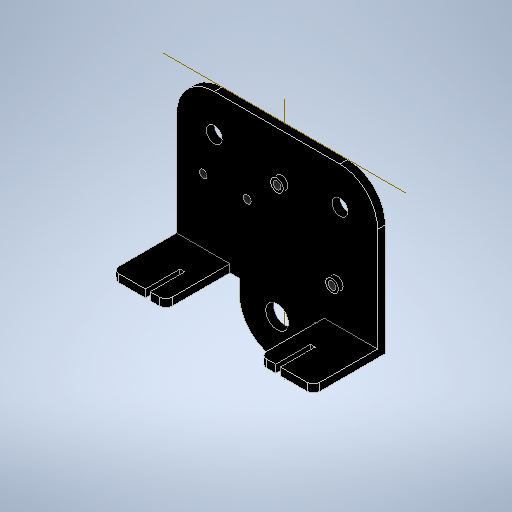
# Autodesk Inventor part: Extruder Plate
Saved by Autodesk Inventor 2025 (Build 290162000, 162)
## iProperties
Manager: J. Wilburn
Created: 2025-03-12
Part Number: Extruder Plate
Material: Aluminum 6061
Document SubType Name: Modeling
Designer: MAL16204
Density: 2.7 g/cm^3
Appearance: Anodized - Black
Mass: 26.6308 g
Surface Area: 91.3048 cm^2
Volume: 9.86327 cm^3
Author: Richard Malstrom
Title: Extruder Plate
Subject: Ender 3 Pro Assembly
Autodesk Inventor part; units mm, degrees
ref_plane "YZ Plane" through (0, 0, 0) normal (1, 0, 0) x (0, 1, 0)
ref_plane "XZ Plane" through (0, 0, 0) normal (0, 1, 0) x (-1, 0, 0)
ref_plane "XY Plane" through (0, 0, 0) normal (0, 0, 1) x (1, 0, 0)
sketch "Sketch1" plane through (0, 0, 0) normal (0, 0, 1) x (1, 0, 0)
  line L0 (-20, 0) -> (20, 0)
  line L1 (32, -12) -> (32, -47.5)
  line L2 (0, -64) -> (0, -64)
  line L3 (-32, -47.5) -> (-32, -12)
  arc A0 (-20, 0) -> (-32, -12) centre (-20, -12) ccw
  arc A1 (32, -12) -> (20, 0) centre (20, -12) ccw
  line L4 (-12, -52) -> (-12, -47.5)
  line L5 (-12, -47.5) -> (-32, -47.5)
  line L6 (12, -52) -> (12, -47.5)
  line L7 (12, -47.5) -> (32, -47.5)
  circle A2 centre (0, -52.1) radius 3.6
  line L8 (0, -80.2794) -> (0, 16.2794) projected
  arc A3 (-12, -52) -> (0, -64) centre (0, -52) ccw
  arc A4 (0, -64) -> (12, -52) centre (0, -52) ccw
  point P0 (0, 0)
  point P1 (0, 0)
  point P2 (0, -64)
  dimension "d0" = 64
  dimension "d1" = 64
  dimension "d2" = 12
  dimension "d3" = 47.5
  dimension "d4" = 47.5
  dimension "d5" = 7.2
  dimension "d6" = 52.1
  dimension "d8" = 12
  dimension "d9" = 12
  dimension "d10" = 12
  constraints: 16 end point, 8 point on circle, 8 tangent, 5 centre point, 2 equal radius, 2 parallel, 1 coincident, 1 horizontal, 1 midpoint, 1 perpendicular, 1 point on line
  measures "d0" distance from line of point (0, 0) L2
  measures "d1" distance between parallel lines of L1 L3
  measures "d2" radius of A0
  measures "d3" distance between parallel lines of L0 L5
  measures "d4" distance between parallel lines of L0 L7
  measures "d5" diameter of A2
  measures "d6" distance of point (0, 0) A2.centre
  measures "d8" distance between parallel lines of L8 L4
  measures "d9" distance between parallel lines of L6 L8
  measures "d10" radius of A3
extrude "Extrusion1" add sketch "Sketch1" along normal blind 2.5 contours L0 L8 A2 A3 L4 L5 L3 A0 | L0 A1 L1 L7 L6 A4 L8 A2
sketch "Sketch2" plane through (0, 0, 2.5) normal (0, 0, 1) x (1, 0, 0)
  line L0 (-32, -47.5) -> (-15, -47.5)
  line L1 (-15, -47.5) -> (-15, -45)
  line L2 (-15, -45) -> (-32, -45)
  line L3 (-32, -45) -> (-32, -47.5)
  line L4 (32, -47.5) -> (32, -12) projected
  line L5 (32, -47.5) -> (15, -47.5)
  line L6 (15, -47.5) -> (15, -45)
  line L7 (15, -45) -> (32, -45)
  line L8 (32, -45) -> (32, -47.5)
  point P0 (0, 0)
  point P1 (-12, -47.5)
  point P2 (12, -47.5)
  point P3 (32, -45)
  point P4 (15, -46.25)
  point P5 (-15, -46.25)
  dimension "d13" = 2.5
  dimension "d17" = 30
  dimension "d18" = 2.5
  constraints: 16 end point, 4 parallel, 2 horizontal, 2 midpoint, 2 perpendicular, 1 collinear, 1 point on line
  measures "d13" distance of L1.end L0.end
  measures "d17" distance of point (15, -46.25) point (-15, -46.25)
  measures "d18" distance between parallel lines of L5 L7
extrude "Extrusion2" add sketch "Sketch2" along normal blind 20.4
sketch "Sketch3" plane through (15, -45, 2.5) normal (0, 1, 0) x (1, 0, 0)
  line L0 (0, -20.4) -> (17, -20.4) projected
  line L1 (6.5, -20.4) -> (5, -20.4)
  line L2 (5, -20.4) -> (5, -9.4)
  line L3 (5, -9.4) -> (6.5, -9.4)
  line L4 (6.5, -9.4) -> (6.5, -20.4)
  line L5 (-3, 2.5) -> (17, 2.5) projected
  line L6 (-30, -20.4) -> (-47, -20.4) projected
  line L7 (-35, -20.4) -> (-36.5, -20.4)
  line L8 (-36.5, -20.4) -> (-36.5, -9.4)
  line L9 (-36.5, -9.4) -> (-35, -9.4)
  line L10 (-35, -9.4) -> (-35, -20.4)
  line L11 (-47, 2.5) -> (-27, 2.5) projected
  line L12 (0, 0) -> (0, -20.4) projected
  point P0 (-15, 2.5)
  point P1 (5, -14.9)
  point P2 (5, -20.4)
  dimension "d19" = 1.5
  dimension "d20" = 11.9
  dimension "d21" = 1.5
  dimension "d22" = 11.9
  dimension "d23" = 40
  dimension "d24" = 5
  constraints: 16 end point, 4 parallel, 2 horizontal, 2 perpendicular, 2 point on line, 1 midpoint
  measures "d19" distance of L2.end L3.end
  measures "d20" distance between parallel lines of L5 L3
  measures "d21" distance of L8.end L9.end
  measures "d22" distance between parallel lines of L11 L9
  measures "d23" distance between parallel lines of L10 L2
  measures "d24" distance from line of L12 point (5, -14.9)
extrude "Extrusion3" cut sketch "Sketch3" against normal through all
fillet "Fillet1" radius 2 4 edges at (32, -46.25, 22.9) (15, -46.25, 22.9) (-15, -46.25, 22.9) (-32, -46.25, 22.9)
sketch "Sketch4" plane through (0, 0, 0) normal (0, 0, -1) x (-1, 0, 0)
  line L0 (-20, 0) -> (20, 0) projected
  line L1 (-32, -47.5) -> (-32, -12) projected
  line L2 (0, -76.8) -> (0, 12.8) projected
  point P0 (0, 0)
  point P1 (-20, -11.9)
  point P2 (20, -11.9)
  dimension "d28" = 11.9
  dimension "d30" = 20
  dimension "d31" = 20
  constraints: 1 horizontal alignment
  measures "d28" distance from line of L0 point (-20, -11.9)
  measures "d30" distance from line of L2 point (-20, -11.9)
  measures "d31" distance from line of point (20, -11.9) L2
hole "Hole1" at (20, -11.9, 0) at (-20, -11.9, 0) direction (0, 0, 1) diameter 5 end through all
sketch "Sketch5" plane through (0, 0, 0) normal (0, 0, -1) x (-1, 0, 0)
  line L0 (0, -76.8) -> (0, 12.8) projected
  line L1 (-20, 0) -> (20, 0) projected
  point P0 (0, 0)
  point P1 (-19, -33.25)
  point P2 (-1.5, -14.35)
  dimension "d39" = 19
  dimension "d40" = 33.25
  dimension "d41" = 1.5
  dimension "d42" = 14.35
  measures "d39" distance from line of L0 point (-19, -33.25)
  measures "d40" distance from line of L1 point (-19, -33.25)
  measures "d41" distance from line of L0 point (-1.5, -14.35)
  measures "d42" distance from line of L1 point (-1.5, -14.35)
hole "Hole2" at (19, -33.25, 0) at (1.5, -14.35, 0) direction (0, 0, 1) diameter 2.459 end through all thread size "M3x0.5" class "6H" standard "ISO Metric profile"
sketch "Sketch6" plane through (0, 0, 0) normal (0, 0, -1) x (-1, 0, 0)
  line L0 (-20, 0) -> (20, 0) projected
  line L1 (0, -76.8) -> (0, 12.8) projected
  point P0 (0, 0)
  point P1 (9.5, -24.45)
  point P2 (23.5, -24.45)
  dimension "d50" = 24.45
  dimension "d51" = 9.5
  dimension "d52" = 23.5
  constraints: 1 horizontal alignment
  measures "d50" distance from line of L0 point (9.5, -24.45)
  measures "d51" distance from line of L1 point (9.5, -24.45)
  measures "d52" distance from line of L1 point (23.5, -24.45)
hole "Hole3" at (-9.5, -24.45, 0) at (-23.5, -24.45, 0) direction (0, 0, 1) diameter 2.459 end through all thread size "M3x0.5" class "6H" standard "ISO Metric profile"
sketch "Sketch7" plane through (0, 0, 0) normal (0, 0, -1) x (-1, 0, 0)
  circle A0 centre (9.5, -24.45) radius 1.2295 projected
  circle A1 centre (9.5, -24.45) radius 2.7
  circle A2 centre (23.5, -24.45) radius 1.2295 projected
  circle A3 centre (23.5, -24.45) radius 2.7
  point P0 (0, 0)
  dimension "d60" = 5.4
  dimension "d61" = 5.4
  constraints: 2 centre point, 2 coincident
  measures "d60" diameter of A1
  measures "d61" diameter of A3
extrude "Extrusion4" add sketch "Sketch7" along normal blind 4.5
sketch "Sketch8" plane through (0, 0, 2.5) normal (0, 0, 1) x (1, 0, 0)
  circle A0 centre (1.5, -14.35) radius 1.2295 projected
  circle A1 centre (1.5, -14.35) radius 2
  circle A2 centre (19, -33.25) radius 1.2295 projected
  circle A3 centre (19, -33.25) radius 2
  point P0 (0, 0)
  dimension "d64" = 4
  dimension "d65" = 4
  constraints: 2 centre point, 2 coincident
  measures "d64" diameter of A1
  measures "d65" diameter of A3
extrude "Extrusion5" add sketch "Sketch8" along normal blind 1.5
body "Solid1"
